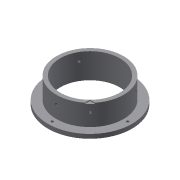
# Autodesk Inventor part: collar_paper
Saved by Autodesk Inventor 2017 (Build 210142000, 142)
## iProperties
Created: 2015-08-14
Part Number: collar_paper
Material: Generic
Document SubType Name: Modeling
Designer: Dave
Density: 1 g/cm^3
Appearance: Default
Author: Dave
Autodesk Inventor part; units mm, degrees
sketch "Sketch1" plane through (0, 0, 0) normal (0, 1, 0) x (-1, 0, 0)
  circle A0 centre (0, 0) radius 63.5
  dimension "d0" = 127
  constraints: 1 centre point, 1 coincident
  measures "d0" diameter of A0
extrude "Extrusion1" add sketch "Sketch1" along normal blind 38.1
sketch "Sketch2" plane through (0, 38.1, 0) normal (0, 1, 0) x (1, 0, 0)
  circle A0 centre (0, 0) radius 63.5 projected
  circle A1 centre (0, 0) radius 45.085
  dimension "d3" = 90.17
  constraints: 1 centre point, 1 coincident
  measures "d3" diameter of A1
hole "centralHole" at (0, 38.1, 0) direction (0, -1, 0) diameter 90.17 end through all
sketch "Sketch3" plane through (0, 38.1, 0) normal (0, 1, 0) x (1, 0, 0)
  circle A0 centre (0, 0) radius 63.5 projected
  circle A1 centre (0, 0) radius 50.8
  dimension "d11" = 101.6
  constraints: 1 centre point, 1 coincident
  measures "d11" diameter of A1
extrude "Extrusion2" cut sketch "Sketch3" against normal blind 31.75
sketch "Sketch4" plane through (0, 6.35, 0) normal (0, 1, 0) x (1, 0, 0)
  circle A0 centre (0, 0) radius 50.8
  circle A1 centre (0, 57.15) radius 2.814303
  dimension "d14" = 57.15
  constraints: 1 centre point
  measures "d14" distance of A0.centre A1.centre
hole "Hole2" at (0, 6.35, -57.15) direction (0, -1, 0) diameter 3.81 end through all
pattern_circular "Circular Pattern1" count 4 over 360 about axis through (0, -10, 0) along (0, 1, 0) of "Hole2"
ref_plane "Work Plane1" through (0, 0, 50.8) normal (0, 0, 1) x (1, 0, 0)
sketch "Sketch5" plane through (0, 0, 50.8) normal (0, 0, 1) x (1, 0, 0)
  circle A0 centre (0, 25.4) radius 3.127107
  line L0 (50.8, 38.1) -> (-50.8, 38.1)
  point P0 (0, 0)
  dimension "d26" = 12.7
  constraints: 1 centre point
  measures "d26" distance from line of A0.centre L0
hole "Hole3" at (0, 25.4, 50.8) direction (0, 0, -1) diameter 3.9624 depth 25.4 tip angle 118 thread size "10-32 UNF" class "2B" standard "ANSI Unified Screw Threads"
pattern_circular "Circular Pattern2" count 3 over 360 about axis through (0, -10, 0) along (0, 1, 0) of "Hole3"
ref_plane "Work Plane3" through (35.921024, 0, 35.921024) normal (0.7071068, 0, 0.7071068) x (0, 1, 0)
ref_plane "Work Plane2" through (0, 0, 0) normal (0.7071068, 0, 0.7071068) x (0, 1, 0)
sketch "Sketch6" plane through (35.921024, 0, 35.921024) normal (0.7071068, 0, 0.7071068) x (0, 1, 0)
  circle A0 centre (25.4, 0) radius 2.162828
  line L0 (38.1, -50.8) -> (38.1, 50.8)
  point P0 (0, 0)
  dimension "d39" = 12.7
  constraints: 1 centre point
  measures "d39" distance from line of A0.centre L0
hole "Hole4" at (35.921024, 25.4, 35.921024) direction (-0.7071068, 0, -0.7071068) diameter 3.9624 depth 25.4 tip angle 118 thread size "10-32 UNF" class "2B" standard "ANSI Unified Screw Threads"
sketch "Sketch7" plane through (0, 38.1, 0) normal (0, 1, 0) x (1, 0, 0)
  circle A0 centre (0, 0) radius 50.8
  circle A1 centre (0, 0) radius 45.085
  line L0 (0, 0) -> (35.921024, -35.921024) construction
  line L1 (0, 0) -> (50.8, 0) construction
  line L2 (31.879909, -31.879909) -> (39.551377, -31.879909)
  line L3 (31.879909, -31.879909) -> (31.879909, -39.551377)
  dimension "d47" = 45
  constraints: 8 end point, 3 point on circle, 1 equal length, 1 horizontal, 1 parallel, 1 perpendicular, 1 point on line, 2 other
  measures "d47" angle of L0 L1
sketch "Sketch7 outline for Extrusion3" plane through (0, 38.1, 0) normal (0, 1, 0) x (1, 0, 0)
  line L0 (39.551377, -31.879909) -> (31.879909, -31.879909)
  arc A0 (31.879909, -39.551377) -> (39.551377, -31.879909) centre (0, 0) ccw
  line L1 (31.879909, -31.879909) -> (31.879909, -39.551377)
extrude "Extrusion3" cut sketch "Sketch7 outline for Extrusion3" against normal blind 1.524
ref_plane "Work Plane7" through (31.879909, 38.1, 39.551377) normal (-0.7071068, 0, -0.7071068) x (0, 1, 0)
sketch "Sketch9" plane through (31.879909, 38.1, 39.551377) normal (-0.7071068, 0, -0.7071068) x (0, 1, 0)
  line L0 (-1.524, 10.849093) -> (-1.524, 0)
  line L1 (-1.524, 0) -> (-1.524, 10.849093)
  line L2 (-1.524, 10.849093) -> (-2.524, 10.849093)
  line L3 (-2.524, 10.849093) -> (-2.524, 0)
  line L4 (-2.524, 0) -> (-1.524, 0)
  point P0 (-38.1, 5.424547)
  dimension "d50" = 1
  constraints: 8 end point, 3 equal length, 1 perpendicular
  measures "d50" distance of L2.end L0.start
extrude "Extrusion4" cut sketch "Sketch9" against normal up to next
body "Solid1"
